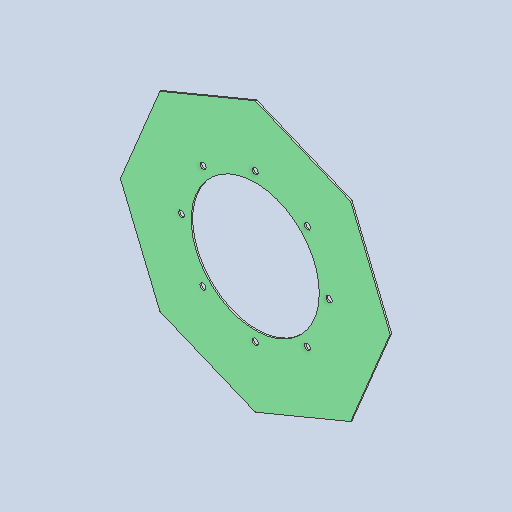
# Autodesk Inventor part: ДМС 101 Барабан торец
Saved by Autodesk Inventor 2024.2 (Build 282272000, 272)
## iProperties
Created: 2024-04-28
Part Number: ДМС 101 Барабан торец
Material: Generic
Document SubType Name: Sheet Metal
Designer: pokla
Density: 1 g/cm^3
Appearance: Default
Sheet Metal Rule: Default
Author: pokla
Autodesk Inventor part; units mm, degrees
ref_plane "YZ Plane" through (0, 0, 0) normal (1, 0, 0) x (0, 1, 0)
ref_plane "XZ Plane" through (0, 0, 0) normal (0, 1, 0) x (-1, 0, 0)
ref_plane "XY Plane" through (0, 0, 0) normal (0, 0, 1) x (1, 0, 0)
sketch "Sketch2" plane through (0, 0, 0) normal (0, 0, 1) x (1, 0, 0)
  line L0 (-193.6378, 193.6378) -> (0, 273.8452)
  line L1 (0, 273.8452) -> (193.6378, 193.6378)
  line L2 (193.6378, 193.6378) -> (273.8452, 0)
  line L3 (273.8452, 0) -> (193.6378, -193.6378)
  line L4 (193.6378, -193.6378) -> (0, -273.8452)
  line L5 (0, -273.8452) -> (-193.6378, -193.6378)
  line L6 (-193.6378, -193.6378) -> (-273.8452, 0)
  line L7 (-273.8452, 0) -> (-193.6378, 193.6378)
  circle A0 centre (0, 0) radius 130
  dimension "d23" = 506
  dimension "d26" = 260
  measures "d23" distance between parallel lines of L6 L2
  measures "d26" diameter of A0
extrude "Plate1" add sketch "Sketch2" against normal blind 3
sketch "Sketch4" plane through (0, 0, 0) normal (0, 0, 1) x (1, 0, 0)
  circle A0 centre (0, 150) radius 6.25
  circle A1 centre (0, 0) radius 130 projected
  dimension "d16" = 12.5
  dimension "d17" = 150
  constraints: 1 centre point, 1 vertical alignment
  measures "d16" diameter of A0
  measures "d17" distance of point (0, 0) A0.centre
extrude "Extrusion1" cut sketch "Sketch4" against normal up to surface (3 mm away) contours A0
pattern_circular "Circular Pattern1" count 8 over 360 about axis through (0, 0, -10) along (0, 0, 1) of "Extrusion1"
equation "\"d23\" = Барабан_габарит_по_кассетам"
equation "\"d26\" = Вал_ось_диаметр_лицо"
equation "\"d15\" = Thickness"
equation "\"BendRadius\" = Thickness"
equation "\"BendReliefWidth\" = Thickness"
equation "\"BendReliefDepth\" = 0.5 * Thickness"
equation "\"CornerReliefSize\" = 4 * Thickness"
equation "\"MinimumRemnant\" = 2 * Thickness"
equation "\"TransitionRadius\" = BendRadius"
equation "\"JacobiRadiusSize\" = BendRadius"
equation "\"GapSize\" = Thickness"
equation "\"Барабан_габарит_по_кассетам\" = 506"
equation "\"Вал_ось_диаметр_лицо\" = 260"
equation "\"Thickness\" = 3"
body "Solid1"
